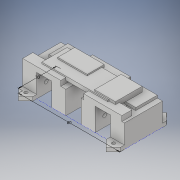
# Autodesk Inventor part: ball-waterfall
Saved by Autodesk Inventor 2017 (Build 210142000, 142)
## iProperties
Created: 2017-03-05
Part Number: ball-waterfall
Material: Generic
Document SubType Name: Modeling
Designer: John
Density: 1 g/cm^3
Appearance: Default
Author: John
Autodesk Inventor part; units mm, degrees
ref_plane "YZ Plane" through (0, 0, 0) normal (1, 0, 0) x (0, 1, 0)
ref_plane "XY Plane" through (0, 0, 0) normal (0, 0, 1) x (1, 0, 0)
sketch "Sketch1" plane through (0, 0, 0) normal (0, 1, 0) x (-1, 0, 0)
  line L0 (0, 0) -> (80, 0) construction
  line L1 (80, 0) -> (80, 30) construction
  line L2 (80, 30) -> (0, 30) construction
  line L3 (0, 30) -> (0, 0) construction
  dimension "d0" = 80
  dimension "d1" = 30
  constraints: 8 end point, 2 parallel, 1 horizontal, 1 perpendicular
  measures "d0" distance of L2.end L1.end
  measures "d1" distance of L1.end L0.end
sketch "Sketch2" plane through (0, 0, 0) normal (0, 1, 0) x (-1, 0, 0)
  line L0 (80, 0) -> (69, 0)
  line L1 (69, 0) -> (69, 30)
  line L2 (69, 30) -> (80, 30)
  line L3 (80, 30) -> (80, 0)
  line L4 (0, 0) -> (11, 0)
  line L5 (11, 0) -> (11, 30)
  line L6 (11, 30) -> (0, 30)
  line L7 (0, 30) -> (0, 0)
  line L8 (57, 0) -> (46, 0)
  line L9 (46, 0) -> (46, 30)
  line L10 (46, 30) -> (57, 30)
  line L11 (57, 30) -> (57, 0)
  line L12 (34, 0) -> (23, 0)
  line L13 (23, 0) -> (23, 30)
  line L14 (23, 30) -> (34, 30)
  line L15 (34, 30) -> (34, 0)
  line L16 (69, 15) -> (57, 15) construction
  line L17 (46, 15) -> (34, 15) construction
  line L18 (23, 15) -> (11, 15) construction
  line L19 (71, 2) -> (78, 2)
  line L20 (78, 2) -> (78, 28)
  line L21 (78, 28) -> (71, 28)
  line L22 (71, 28) -> (71, 2)
  line L23 (55, 2) -> (48, 2)
  line L24 (48, 2) -> (48, 28)
  line L25 (48, 28) -> (55, 28)
  line L26 (55, 28) -> (55, 2)
  line L27 (32, 2) -> (25, 2)
  line L28 (25, 2) -> (25, 28)
  line L29 (25, 28) -> (32, 28)
  line L30 (32, 28) -> (32, 2)
  line L31 (9, 28) -> (9, 2)
  line L32 (9, 2) -> (2, 2)
  line L33 (2, 2) -> (2, 28)
  line L34 (2, 28) -> (9, 28)
  dimension "d2" = 11
  dimension "d3" = 30
  dimension "d4" = 11
  dimension "d6" = 11
  dimension "d8" = 11
  dimension "d9" = 80
  dimension "d10" = 2
  dimension "d11" = 2
  dimension "d12" = 2
  dimension "d13" = 2
  constraints: 70 end point, 16 parallel, 8 perpendicular, 6 collinear, 6 midpoint, 4 horizontal, 2 point on line, 12 other
  measures "d2" distance of L1.end L2.end
  measures "d3" distance of L0.end L1.end
  measures "d4" distance of L6.end L5.end
  measures "d6" distance of L9.end L10.end
  measures "d8" distance of L13.end L14.end
  measures "d9" distance between parallel lines of L7 L3
  measures "d10" distance between parallel lines of L0 L19
  measures "d11" distance between parallel lines of L11 L26
  measures "d12" distance between parallel lines of L15 L30
  measures "d13" distance between parallel lines of L5 L31
extrude "Extrusion1" add sketch "Sketch2" along normal blind 15
sketch "Sketch3" plane through (0, 15, 0) normal (0, 1, 0) x (1, 0, 0)
  line L0 (-69, 0) -> (-80, 0) projected
  line L1 (-80, 0) -> (-69, 0)
  line L2 (-69, 0) -> (-69, -30)
  line L3 (-69, -30) -> (-80, -30)
  line L4 (-80, -30) -> (-80, 0)
  line L5 (-57, 0) -> (-46, 0)
  line L6 (-46, 0) -> (-46, -30)
  line L7 (-46, -30) -> (-57, -30)
  line L8 (-57, -30) -> (-57, 0)
  line L9 (-34, 0) -> (-23, 0)
  line L10 (-23, 0) -> (-23, -30)
  line L11 (-23, -30) -> (-34, -30)
  line L12 (-34, -30) -> (-34, 0)
  line L13 (-11, 0) -> (0, 0)
  line L14 (0, 0) -> (0, -30)
  line L15 (0, -30) -> (-11, -30)
  line L16 (-11, -30) -> (-11, 0)
  dimension "d16" = 30
  dimension "d19" = 23
  constraints: 32 end point, 2 horizontal, 2 parallel, 1 collinear, 1 perpendicular, 26 other
  measures "d16" distance of L1.end L2.end
  measures "d19" distance of L0.start point (-46, 0)
extrude "Extrusion2" add sketch "Sketch3" along normal blind 3
sketch "Sketch4" plane through (-69, 0, 30) normal (1, 0, 0) x (0, 0, -1)
  circle A0 centre (7.5, 8) radius 1.5
  line L0 (2, 0) -> (28, 0) projected
  line L1 (0, 0) -> (0, 18) construction
  dimension "d26" = 3
  dimension "d28" = 8
  dimension "d29" = 7.5
  constraints: 1 centre point
  measures "d26" diameter of A0
  measures "d28" distance from line of L0 A0.centre
  measures "d29" distance from line of L1 A0.centre
extrude "Extrusion3" cut sketch "Sketch4" against normal blind 3
sketch "Sketch5" plane through (-57, 0, 0) normal (-1, 0, 0) x (0, 0, 1)
  circle A0 centre (22.5, 8) radius 1.5
  line L0 (30, 0) -> (30, 18) projected
  line L1 (2, 0) -> (28, 0) projected
  point P0 (0, 0)
  dimension "d33" = 3
  dimension "d34" = 7.5
  dimension "d35" = 8
  constraints: 1 centre point
  measures "d33" diameter of A0
  measures "d34" distance from line of L0 A0.centre
  measures "d35" distance from line of L1 A0.centre
extrude "Extrusion4" cut sketch "Sketch5" against normal blind 3
sketch "Sketch6" plane through (-46, 0, 30) normal (1, 0, 0) x (0, 0, -1)
  circle A0 centre (22.5, 8) radius 1.5
  line L0 (30, 0) -> (30, 18) projected
  line L1 (2, 0) -> (28, 0) projected
  dimension "d38" = 3
  dimension "d39" = 7.5
  dimension "d40" = 8
  constraints: 1 centre point
  measures "d38" diameter of A0
  measures "d39" distance from line of L0 A0.centre
  measures "d40" distance from line of L1 A0.centre
sketch "Sketch7" plane through (-34, 0, 0) normal (-1, 0, 0) x (0, 0, 1)
  circle A0 centre (7.5, 8) radius 1.5
  line L0 (2, 0) -> (28, 0) projected
  line L1 (0, 0) -> (0, 18) projected
  dimension "d41" = 3
  dimension "d42" = 8
  dimension "d43" = 7.5
  constraints: 1 centre point
  measures "d41" diameter of A0
  measures "d42" distance from line of L0 A0.centre
  measures "d43" distance from line of L1 A0.centre
sketch "Sketch8" plane through (-23, 0, 30) normal (1, 0, 0) x (0, 0, -1)
  circle A0 centre (7.5, 8) radius 1.5
  line L0 (2, 0) -> (28, 0) projected
  line L1 (0, 0) -> (0, 18) projected
  point P0 (30, 0)
  dimension "d44" = 3
  dimension "d45" = 8
  dimension "d46" = 7.5
  constraints: 1 centre point
  measures "d44" diameter of A0
  measures "d45" distance from line of L0 A0.centre
  measures "d46" distance from line of L1 A0.centre
sketch "Sketch9" plane through (-11, 0, 0) normal (-1, 0, 0) x (0, 0, 1)
  point P0 (0, 0)
sketch "Sketch10" plane through (-11, 0, 0) normal (-1, 0, 0) x (0, 0, 1)
  circle A0 centre (22.5, 8) radius 1.5
  line L0 (30, 0) -> (30, 18) projected
  line L1 (2, 0) -> (28, 0) projected
  point P0 (0, 0)
  dimension "d47" = 3
  dimension "d48" = 7.5
  dimension "d49" = 8
  constraints: 1 centre point
  measures "d47" diameter of A0
  measures "d48" distance from line of L0 A0.centre
  measures "d49" distance from line of L1 A0.centre
extrude "Extrusion5" cut sketch "Sketch6" against normal blind 3
extrude "Extrusion6" cut sketch "Sketch7" against normal blind 3
extrude "Extrusion7" cut sketch "Sketch8" against normal blind 3
extrude "Extrusion8" cut sketch "Sketch10" against normal blind 3
ref_plane "Work Plane1" through (0, 18, 0) normal (0, 1, 0) x (-1, 0, 0)
sketch "Sketch12" plane through (0, 18, 0) normal (0, 1, 0) x (-1, 0, 0)
  line L0 (80, 30) -> (50, 30)
  line L1 (50, 30) -> (50, 22)
  line L2 (50, 22) -> (80, 22)
  line L3 (80, 22) -> (80, 30)
  line L4 (55, 0) -> (25, 0)
  line L5 (25, 0) -> (25, 8)
  line L6 (25, 8) -> (55, 8)
  line L7 (55, 8) -> (55, 0)
  line L8 (32, 2) -> (32, 28) projected
  line L9 (32, 22) -> (2, 22)
  line L10 (2, 22) -> (2, 30)
  line L11 (2, 30) -> (32, 30)
  line L12 (32, 30) -> (32, 22)
  point P0 (0, 0)
  dimension "d59" = 30
  dimension "d60" = 8
  dimension "d61" = 30
  dimension "d62" = 8
  dimension "d63" = 30
  constraints: 24 end point, 6 parallel, 3 horizontal, 3 perpendicular, 3 point on line
  measures "d59" distance of L2.end L1.end
  measures "d60" distance of L1.end L0.end
  measures "d61" distance of L5.end L6.end
  measures "d62" distance of L4.end L5.end
  measures "d63" distance of L10.end L11.end
sketch "Sketch13" plane through (0, 18, 0) normal (0, 1, 0) x (-1, 0, 0)
  line L0 (74.3573, 0) -> (62.3573, 0)
  line L1 (62.3573, 0) -> (62.3573, 15)
  line L2 (62.3573, 15) -> (74.3573, 15)
  line L3 (74.3573, 15) -> (74.3573, 0)
  line L4 (48, 12) -> (36, 12)
  line L5 (36, 12) -> (36, 21)
  line L6 (36, 21) -> (48, 21)
  line L7 (48, 21) -> (48, 12)
  line L8 (0, 0) -> (11, 0) projected
  line L9 (4, 0) -> (17, 0)
  line L10 (17, 0) -> (17, 17)
  line L11 (17, 17) -> (4, 17)
  line L12 (4, 17) -> (4, 0)
  dimension "d64" = 12
  dimension "d65" = 15
  dimension "d66" = 12
  dimension "d67" = 13
  dimension "d68" = 17
  constraints: 24 end point, 6 parallel, 3 horizontal, 3 perpendicular, 1 point on line
  measures "d64" distance of L1.end L2.end
  measures "d65" distance of L0.end L1.end
  measures "d66" distance of L5.end L6.end
  measures "d67" distance of L11.end L10.end
  measures "d68" distance of L10.end L9.end
extrude "Extrusion9" add sketch "Sketch13" along normal blind 2
extrude "Extrusion10" add sketch "Sketch12" along normal blind 4
sketch "Sketch14" plane through (0, 20, 0) normal (0, 1, 0) x (1, 0, 0)
  line L0 (-65, -4) -> (-41.7529, -4)
  line L1 (-41.7529, -4) -> (-41.7529, -17.4715)
  line L2 (-41.7529, -17.4715) -> (-65, -17.4715)
  line L3 (-65, -17.4715) -> (-65, -4)
  line L4 (-12, -25) -> (-28.5, -25)
  line L5 (-28.5, -25) -> (-28.5, -4)
  line L6 (-28.5, -4) -> (-12, -4)
  line L7 (-12, -4) -> (-12, -25)
  point P0 (0, 0)
  dimension "d73" = 16.5
  constraints: 16 end point, 4 parallel, 2 horizontal, 2 perpendicular, 1 point on line
  measures "d73" distance of L5.end L6.end
extrude "Extrusion11" add sketch "Sketch14" along normal blind 4
sketch "Sketch15" plane through (0, 20, 0) normal (0, 1, 0) x (1, 0, 0)
  line L0 (-69, -30) -> (-69, -22) projected
  line L1 (-69, -26) -> (-17, -26)
  line L2 (-17, -26) -> (-17, -6)
  line L3 (-17, -6) -> (-69, -6)
  line L4 (-69, -6) -> (-69, -26)
  point P0 (0, 0)
  dimension "d76" = 52
  dimension "d77" = 20
  constraints: 8 end point, 2 parallel, 1 horizontal, 1 midpoint, 1 perpendicular
  measures "d76" distance of L3.end L2.end
  measures "d77" distance of L2.end L1.end
extrude "Extrusion12" add sketch "Sketch15" along normal blind 3
sketch "Sketch16" plane through (0, 0, 0) normal (0, 1, 0) x (-1, 0, 0)
  line L0 (69, 30) -> (80, 30) projected
  line L1 (80, 30) -> (80, 33)
  line L2 (69, 30) -> (69, 33)
  line L3 (69, 33) -> (74.8182, 38.4908)
  line L4 (74.8182, 38.4908) -> (80, 33)
  circle A0 centre (74.5, 33) radius 1.25
  line L5 (74.5, 33) -> (80, 33) construction
  line L6 (74.5, 33) -> (69, 33) construction
  line L7 (11, 30) -> (11, 33)
  line L8 (0, 30) -> (0, 33)
  line L9 (11, 33) -> (5.5, 38.8095)
  line L10 (5.5, 38.8095) -> (0, 33)
  circle A1 centre (5.5, 33) radius 1.25
  line L11 (5.5, 33) -> (11, 33) construction
  line L12 (5.5, 33) -> (0, 33) construction
  line L13 (80, 15) -> (0, 15) construction
  line L14 (69, 0) -> (80, 0)
  line L15 (80, 0) -> (80, -3)
  line L16 (69, 0) -> (69, -3)
  line L17 (69, -3) -> (74.8182, -8.4908)
  line L18 (74.8182, -8.4908) -> (80, -3)
  circle A2 centre (74.5, -3) radius 1.25
  line L19 (74.5, -3) -> (80, -3) construction
  line L20 (74.5, -3) -> (69, -3) construction
  line L21 (11, 0) -> (11, -3)
  line L22 (0, 0) -> (0, -3)
  line L23 (11, -3) -> (5.5, -8.8095)
  line L24 (5.5, -8.8095) -> (0, -3)
  circle A3 centre (5.5, -3) radius 1.25
  line L25 (5.5, -3) -> (11, -3) construction
  line L26 (5.5, -3) -> (0, -3) construction
  line L27 (80, 0) -> (69, 0) projected
  line L28 (80, 0) -> (69, 0)
  line L29 (11, 0) -> (0, 0)
  line L30 (4, 0) -> (17, 0) projected
  line L31 (11, 30) -> (0, 30)
  dimension "d80" = 3
  dimension "d81" = 3
  dimension "d82" = 8
  dimension "d83" = 2.5
  dimension "d84" = 3
  dimension "d85" = 3
  dimension "d86" = 3
  dimension "d87" = 8
  dimension "d88" = 2.5
  constraints: 58 end point, 10 symmetric about line, 4 centre point, 4 vertical, 3 equal length, 2 collinear, 1 horizontal, 1 parallel, 1 perpendicular, 2 other
  measures "d80" distance of L0.end L1.end
  measures "d81" distance of L0.start L2.end
  measures "d82" distance of L2.end L3.end
  measures "d83" diameter of A0
  measures "d84" distance from line of L0 L5.start
  measures "d85" distance of L7.start L7.end
  measures "d86" distance of L8.start L8.end
  measures "d87" distance of L7.end L9.end
  measures "d88" diameter of A1
extrude "Extrusion14" add sketch "Sketch16" along normal blind 3
equation "\"d11\" = d10"
equation "\"d12\" = d10"
equation "\"d13\" = d10"
equation "\"d81\" = d80"
equation "\"d84\" = d81"
equation "\"d85\" = d86"
equation "\"d86\" = d84"
equation "\"d87\" = d82"
body "Solid1"
